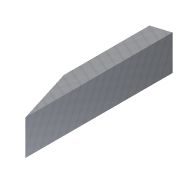
# Autodesk Inventor part: ball shoot
Saved by Autodesk Inventor 2011 (Build 150239000, 239)
## iProperties
Created: 2014-09-14
Part Number: ball shoot
Document SubType Name: Modeling
Designer: Family Room
Density: 1 g/cm^3
Author: Family Room
Autodesk Inventor part; units mm, degrees
ref_plane "YZ Plane" through (0, 0, 0) normal (1, 0, 0) x (0, 1, 0)
ref_plane "XZ Plane" through (0, 0, 0) normal (0, 1, 0) x (-1, 0, 0)
ref_plane "XY Plane" through (0, 0, 0) normal (0, 0, 1) x (1, 0, 0)
sketch "Sketch1" plane through (0, 0, 0) normal (0, 0, 1) x (1, 0, 0)
  line L0 (0, 0) -> (25.4, 0)
  line L1 (25.4, 0) -> (25.4, 50.8)
  line L2 (25.4, 50.8) -> (0, 50.8)
  line L3 (0, 50.8) -> (0, 0)
  line L4 (22.225, 47.625) -> (22.225, 3.175)
  line L5 (22.225, 3.175) -> (3.175, 3.175)
  line L6 (3.175, 3.175) -> (3.175, 47.625)
  line L7 (3.175, 47.625) -> (22.225, 47.625)
  dimension "d0" = 25.4
  dimension "d1" = 50.8
  dimension "d2" = 3.175
  constraints: 16 end point, 4 parallel, 2 perpendicular, 1 horizontal, 3 other
  measures "d0" distance of L2.end L1.end
  measures "d1" distance of L1.end L0.end
  measures "d2" distance between parallel lines of L2 L7
extrude "Extrusion1" add sketch "Sketch1" along normal blind 254
sketch "Sketch4" plane through (0, 50.8, 0) normal (0, 1, 0) x (1, 0, 0)
  line L0 (0, -254) -> (25.4, -254) projected
  line L1 (25.4, 0) -> (25.4, -254) projected
  line L2 (25.4, 0) -> (0, 0) projected
  line L3 (0, 0) -> (0, -254) projected
  line L4 (25.4, -254) -> (-35.2095, -60.0497)
  line L5 (-35.2095, -60.0497) -> (25.4, -41.1092)
  line L6 (25.4, -254) -> (25.4, -41.1092)
  line L7 (0, -49.0467) -> (0, -172.72)
  dimension "d17" = 203.2
  dimension "d18" = 63.5
  constraints: 8 end point, 5 point on line, 1 collinear, 1 perpendicular
  measures "d17" distance of L0.end L4.end
  measures "d18" distance of L4.end L5.end
extrude "Extrusion4" cut sketch "Sketch4" against normal blind 254 contours L3 L4 L0 | L5 L3 L2 L1
body "Solid1"
